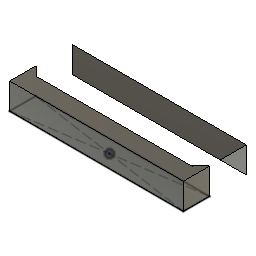
clips v2 (Autodesk Fusion 360 design; units mm, degrees)
Autodesk Fusion 360 part; units mm, degrees
sketch "Esquisse1" plane through (0, 0, 0) normal (0, 0, 1) x (1, 0, 0) in component "clips femelle"
  line L0 (10, 1.5) -> (-10, 1.5)
  line L1 (-10, 1.5) -> (-10, -1.5)
  line L2 (-10, -1.5) -> (10, -1.5)
  line L3 (10, -1.5) -> (10, 1.5)
  line L4 (10, 1.5) -> (-10, -1.5) construction
  line L5 (-10, 1.5) -> (10, -1.5) construction
  dimension "d3" = 20
  dimension "d4" = 3
  constraint horizontal L0
  constraint perpendicular L0 L1
  constraint parallel L0 L2
  constraint parallel L1 L3
  constraint coincident L4 origin
  constraint coincident L5 origin
  measures "d3" distance of L1.end L2.end
  measures "d4" distance of L0.end L1.end
extrude "Extrusion3" add sketch "Esquisse1" along normal blind 1.5 makes body 1 in component "clips femelle"
chamfer "Chanfrein1" distance 1.5 angle 45 1 edges at (0, 1.5, 1.5) on bodies 1 in component "clips femelle"
sketch "Esquisse2" plane through (0, 0, 1.5) normal (0, 0, 1) x (-1, 0, 0) in component "clips femelle"
  line L0 (-10, 0) -> (10, 0)
  line L1 (10, 0) -> (10, 1.5)
  line L2 (10, 1.5) -> (-10, 1.5)
  line L3 (-10, 1.5) -> (-10, 0)
extrude "Extrusion4" add sketch "Esquisse2" along normal blind 1.5 bodies 1 in component "clips femelle"
extrude "Extrusion5" add 1 faces at (3.3333, 0, 2) along direction (0, 1, 0) blind 1.5 on bodies 1 bodies 1 in component "clips femelle"
chamfer "Chanfrein2" distance 1.5 angle 45 1 edges at (0, 1.5, 1.5) on bodies 1 in component "clips femelle"
sketch "Esquisse3" plane through (0, 0, 3) normal (0, 0, 1) x (-1, 0, 0) in component "clips femelle"
  line L0 (-10, 1.5) -> (-10, -1.5)
  line L1 (-10, -1.5) -> (10, -1.5)
  line L2 (10, -1.5) -> (10, 1.5)
  line L3 (10, 1.5) -> (-10, 1.5)
  line L4 (10, -1.5) -> (-10, -1.5)
  line L5 (-10, -1.5) -> (-10, -1)
  line L6 (-10, -1) -> (10, -1)
  line L7 (10, -1) -> (10, -1.5)
  dimension "d17" = 0.5
  constraint perpendicular L4 L5
  constraint parallel L4 L6
  constraint parallel L5 L7
  constraint coincident L0.end L1.start
  constraint perpendicular L0 L4
  constraint coincident L1.end L2.start
  measures "d17" distance of L1.end L6.end
extrude "Extrusion6" cut sketch "Esquisse3" against normal blind 0.5 contours L0 L1 L2 L4 L5 L6 L7 bodies 1 in component "clips femelle"
chamfer "Chanfrein3" distance 0.5 angle 45 1 edges at (0, 1, 3) on bodies 1 in component "clips femelle"
sketch "Esquisse4" plane through (0, 0, 0) normal (0, 0, 1) x (1, 0, 0) in component "clips femelle"
  line L0 (10, 1.5) -> (8.5, 1.5)
  line L1 (8.5, 1.5) -> (8.5, -1.5)
  line L2 (8.5, -1.5) -> (10, -1.5)
  line L3 (10, -1.5) -> (10, 1.5)
  point P0 (10, 1.5)
  dimension "d31" = 1.5
  dimension "d32" = 3
  constraint perpendicular L0 L1
  constraint parallel L0 L2
  constraint parallel L1 L3
  constraint coincident P0 L0.start
  measures "d31" distance of P0 L0.end
  measures "d32" distance of P0 L2.end
extrude "Extrusion7" add sketch "Esquisse4" along normal blind 3 bodies 1 in component "clips femelle"
chamfer "Chanfrein5" distance 1.45 angle 45 1 edges at (8.5, 1.5, 1.5) on bodies 1 in component "clips femelle"
sketch "Esquisse8" plane through (0, -1.5, 0) normal (0, -1, 0) x (1, 0, 0) in component "clips femelle"
  line L0 (10, 3) -> (-10, 3)
  line L1 (-10, 3) -> (-10, 0)
  line L2 (-10, 0) -> (10, 0)
  line L3 (10, 0) -> (10, 3)
  line L4 (-10, 0) -> (-10, 3)
  line L5 (-10, 3) -> (-8.5, 3)
  line L6 (-8.5, 3) -> (-8.5, 0)
  line L7 (-8.5, 0) -> (-10, 0)
  dimension "d44" = 1.5
  constraint perpendicular L4 L5
  constraint parallel L4 L6
  constraint parallel L5 L7
  constraint coincident L0.end L1.start
  constraint coincident L1.end L2.start
  measures "d44" distance of L1.end L6.end
extrude "Extrusion10" add sketch "Esquisse8" against normal blind 3 contours L0 L1 L2 L4 L5 L6 L7 bodies 1 in component "clips femelle"
chamfer "Chanfrein6" distance 1.45 angle 45 1 edges at (-8.5, 1.5, 1.5) on bodies 1 in component "clips femelle"
sketch "Esquisse1 (2)" plane through (0, 0, 0) normal (0, 0, 1) x (1, 0, 0) in component "clips male"
  line L0 (10, 5.75) -> (-10, 5.75)
  line L1 (-10, 5.75) -> (-10, 4.25)
  line L2 (-10, 4.25) -> (10, 4.25)
  line L3 (10, 4.25) -> (10, 5.75)
  line L4 (10, 5.75) -> (-10, 4.25) construction
  line L5 (-10, 5.75) -> (10, 4.25) construction
  point P0 (0, 5)
  dimension "d21" = 20
  dimension "d22" = 1.5
  constraint horizontal L0
  constraint perpendicular L0 L1
  constraint parallel L0 L2
  constraint parallel L1 L3
  constraint coincident L4 P0
  constraint coincident L5 P0
  measures "d21" distance of L1.end L2.end
  measures "d22" distance of L0.end L1.end
extrude "Extrusion1" add sketch "Esquisse1 (2)" along normal blind 3 separate body makes body 2 in component "clips male"
chamfer "Chanfrein3'" distance 1.5 angle 45 1 edges at (10, 4.25, 1.5) on bodies 2 in component "clips male"
chamfer "Chanfrein4" distance 1.5 angle 45 1 edges at (-10, 4.25, 1.5) on bodies 2 in component "clips male"
chamfer "Chanfrein5'" distance 1.5 angle 45 1 edges at (0, 4.25, 3) on bodies 2 in component "clips male"
chamfer "Chanfrein6'" distance 1.5 angle 45 1 edges at (0, 4.25, 0) on bodies 2 in component "clips male"
component "clips femelle" placed x (1, 0, 0) y (0, 1, 0) z (0, 0, 1) at (0, 0, 0)
component "clips male" placed x (1, 0, 0) y (0, 1, 0) z (0, 0, 1) at (0, 0, 0)
equation "Longueur = 20 mm"
equation "largeur = 3 mm"
equation "d3 = Longueur"
equation "d4 = largeur"
equation "d9 = largeur / 2"
equation "d11 = largeur / 2"
equation "d12 = largeur / 2"
equation "d14 = largeur / 2"
equation "d16 = largeur / 2"
equation "d17 = largeur / 6"
equation "d18 = -largeur / 6"
equation "d20 = largeur / 6"
equation "d21 = Longueur"
equation "d22 = largeur / 2"
equation "d23 = largeur"
equation "d27 = largeur / 2"
equation "d28 = largeur / 2"
equation "d29 = largeur / 2"
equation "d30 = largeur / 2"
equation "d31 = largeur / 2"
equation "d32 = largeur"
equation "d33 = largeur"
equation "d43 = largeur / 2 - 0.05 mm"
equation "d44 = largeur / 2"
equation "d45 = -largeur"
equation "d47 = largeur / 2 - 0.05 mm"
